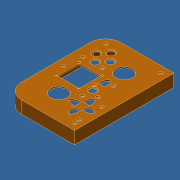
# Autodesk Inventor part: P1704_018_hautManette
Saved by Autodesk Inventor 2019 (Build 230136000, 136)
## iProperties
Created: 2019-05-28
Part Number: P1704_018_hautManette
Project: Nom Projet
Material: .
Description: Nom pièce
Document SubType Name: Modeling
Designer: Adel.KAHRIMANOVIC
Authority: brut Ø
Density: 0.001 g/cm^3
Appearance: Orange
Material number: ---
Author: Adel.KAHRIMANOVIC
Autodesk Inventor part; units mm, degrees
ref_plane "Plan YZ" through (0, 0, 0) normal (1, 0, 0) x (0, 1, 0)
ref_plane "Plan XZ" through (0, 0, 0) normal (0, 1, 0) x (-1, 0, 0)
ref_plane "Plan XY" through (0, 0, 0) normal (0, 0, 1) x (1, 0, 0)
sketch "Esquisse1" plane through (0, 0, 0) normal (0, 0, 1) x (1, 0, 0)
  line L0 (55, 80) -> (55, -80)
  line L1 (-55, -80) -> (-55, 80)
  line L2 (-55, 80) -> (55, -80) construction
  line L3 (55, 80) -> (-55, -80) construction
  line L4 (0, 0) -> (-55, 0) construction
  arc A0 (-55, -55) -> (-30, -80) centre (-30, -55) ccw
  line L5 (-30, -80) -> (55, -80)
  line L6 (-30, -80) -> (-30, -55) construction
  line L7 (55, 80) -> (-30, 80)
  arc A1 (-30, 80) -> (-55, 55) centre (-30, 55) ccw
  line L8 (-30, 55) -> (-30, 80) construction
  line L9 (-83.2132, 0) -> (78.0355, 0) projected
  line L10 (0, -119.2487) -> (0, 119.2487) projected
  dimension "d2" = 160
  dimension "d3" = 110
  dimension "d4" = 25
  dimension "d5" = 25
  constraints: 18 end point, 4 midpoint, 4 point on circle, 3 horizontal, 2 centre point, 2 parallel, 2 point on line, 2 tangent, 2 vertical, 1 collinear, 1 perpendicular
  measures "d2" distance of L0.start L0.end
  measures "d3" distance of L0.end L1.start
  measures "d4" distance of L5.start L6.end
  measures "d5" distance of L8.start L7.end
extrude "Extrusion1" add sketch "Esquisse1" along normal blind 22
sketch "Esquisse6" plane through (0, 0, 0) normal (0, 0, -1) x (-1, 0, 0)
  line L0 (-52.5, 77.5) -> (-52.5, -77.5)
  line L1 (-52.5, -77.5) -> (30, -77.5)
  line L2 (-52.5, 77.5) -> (30, 77.5)
  arc A0 (52.5, 55) -> (30, 77.5) centre (30, 55) ccw
  line L3 (52.5, 55) -> (52.5, -55)
  arc A1 (30, -77.5) -> (52.5, -55) centre (30, -55) ccw
  line L4 (-55, 80) -> (30, 80) projected
  line L5 (-55, -80) -> (-55, 80) projected
  line L6 (30, -80) -> (-55, -80) projected
  line L7 (55, 55) -> (55, -55) projected
  line L8 (30, -239.7653) -> (30, 84.7653) construction
  arc A2 (55, 55) -> (30, 80) centre (30, 55) ccw projected
  line L9 (-55, -80) -> (-55, 80) projected
  line L10 (30, -80) -> (-55, -80) projected
  arc A3 (30, -80) -> (55, -55) centre (30, -55) ccw projected
  line L11 (55, 55) -> (55, -55) projected
  arc A4 (55, 55) -> (30, 80) centre (30, 55) ccw projected
  line L12 (-55, 80) -> (30, 80) projected
  point P0 (0, 0)
  dimension "d8" = 2.5
  dimension "d9" = 2.5
  dimension "d10" = 2.5
  dimension "d11" = 2.5
  constraints: 10 end point, 4 point on circle, 4 tangent, 3 vertical, 2 centre point, 2 point on line, 1 horizontal, 1 midpoint, 1 perpendicular
  measures "d8" distance between parallel lines of L4 L2
  measures "d9" distance between parallel lines of L5 L0
  measures "d10" distance between parallel lines of L6 L1
  measures "d11" distance between parallel lines of L7 L3
extrude "Extrusion2" cut sketch "Esquisse6" against normal blind 2
sketch "Esquisse7" plane through (0, 0, 0) normal (0, 0, -1) x (-1, 0, 0)
  line L0 (-50, 75) -> (-50, -75)
  line L1 (-50, -75) -> (30, -75)
  line L2 (50, 55) -> (50, -55)
  line L3 (-50, 75) -> (30, 75)
  arc A0 (50, 55) -> (30, 75) centre (30, 55) ccw
  arc A1 (30, -75) -> (50, -55) centre (30, -55) ccw
  line L4 (30, 77.5) -> (-52.5, 77.5) projected
  line L5 (-52.5, 77.5) -> (-52.5, -77.5) projected
  line L6 (-52.5, -77.5) -> (30, -77.5) projected
  line L7 (52.5, -55) -> (52.5, 55) projected
  line L8 (30, 77.5) -> (30, 105.4816) construction
  point P0 (0, 0)
  dimension "d14" = 2.5
  dimension "d15" = 2.5
  dimension "d16" = 2.5
  dimension "d17" = 2.5
  constraints: 10 end point, 4 point on circle, 4 tangent, 3 vertical, 2 centre point, 2 point on line, 1 horizontal, 1 perpendicular
  measures "d14" distance between parallel lines of L3 L4
  measures "d15" distance between parallel lines of L5 L0
  measures "d16" distance between parallel lines of L6 L1
  measures "d17" distance between parallel lines of L7 L2
extrude "Extrusion3" cut sketch "Esquisse7" against normal blind 20
sketch "Esquisse8" plane through (0, 0, 22) normal (0, 0, 1) x (1, 0, 0)
  line L0 (-35, -17.5) -> (0, -17.5)
  line L1 (0, -17.5) -> (0, 17.5)
  line L2 (0, 17.5) -> (-35, 17.5)
  line L3 (-35, 17.5) -> (-35, -17.5)
  line L4 (-55, 55) -> (-55, -55) projected
  line L5 (-30, -80) -> (55, -80) projected
  line L6 (-13.2667, 17.5) -> (-13.2667, 80) construction
  line L7 (-17.5, -80) -> (-17.5, -17.5) construction
  line L8 (55, 80) -> (-30, 80) projected
  point P0 (0, 0)
  dimension "d20" = 35
  dimension "d21" = 35
  dimension "d24" = 20
  constraints: 12 end point, 3 parallel, 3 point on line, 2 vertical, 1 horizontal, 1 midpoint, 1 perpendicular
  measures "d20" distance of L2.end L0.start
  measures "d21" distance of L1.end L2.end
  measures "d24" distance between parallel lines of L4 L3
extrude "Extrusion4" cut sketch "Esquisse8" against normal through all
sketch "Esquisse9" plane through (0, 0, 22) normal (0, 0, 1) x (1, 0, 0)
  line L0 (-30, -75) -> (50, -75) projected
  line L1 (-50, 55) -> (-50, -55) projected
  point P0 (0, 0)
  point P1 (44.488, -68.904)
  dimension "d47" = 6.096
  dimension "d48" = 94.488
  measures "d47" distance from line of L0 point (44.488, -68.904)
  measures "d48" distance from line of L1 point (44.488, -68.904)
hole "Perçage1" at (44.488, -68.904, 22) direction (0, 0, -1) diameter 3.4 end through all countersink diameter 6.3 countersink angle 90
sketch "Esquisse10" plane through (0, 0, 22) normal (0, 0, 1) x (1, 0, 0)
  line L0 (-30, -75) -> (50, -75) projected
  line L1 (50, -75) -> (50, 75) projected
  line L2 (-50, 55) -> (-50, -55) projected
  point P0 (0, 0)
  point P1 (43.98, 69.78)
  dimension "d49" = 144.78
  dimension "d51" = 93.98
  measures "d49" distance from line of L0 point (43.98, 69.78)
  measures "d51" distance from line of point (43.98, 69.78) L2
hole "Perçage2" at (43.98, 69.78, 22) direction (0, 0, -1) diameter 3.4 end through all countersink diameter 6.3 countersink angle 90
sketch "Esquisse11" plane through (0, 0, 22) normal (0, 0, 1) x (1, 0, 0)
  line L0 (-30, -75) -> (50, -75) projected
  line L1 (-50, 55) -> (-50, -55) projected
  point P0 (0, 0)
  point P1 (-43.904, 1.2)
  dimension "d52" = 76.2
  dimension "d53" = 6.096
  measures "d52" distance from line of L0 point (-43.904, 1.2)
  measures "d53" distance from line of L1 point (-43.904, 1.2)
hole "Perçage3" at (-43.904, 1.2, 22) direction (0, 0, -1) diameter 3.4 end through all countersink diameter 6.3 countersink angle 90
sketch "Esquisse12" plane through (0, 0, 22) normal (0, 0, 1) x (1, 0, 0)
  circle A0 centre (-10, -40) radius 13.25
  line L0 (-30, -80) -> (55, -80) projected
  line L1 (-55, 55) -> (-55, -55) projected
  line L2 (-30, -75) -> (50, -75) projected
  line L3 (-50, 55) -> (-50, -55) projected
  circle A1 centre (15, 40) radius 13.25
  line L4 (50, -75) -> (50, 75) projected
  line L5 (50, 75) -> (-30, 75) projected
  point P0 (0, 0)
  dimension "d58" = 35
  dimension "d59" = 40
  dimension "d60" = 26.5
  dimension "d61" = 26.5
  dimension "d62" = 35
  dimension "d63" = 35
  constraints: 2 centre point
  measures "d58" distance from line of L2 A0.centre
  measures "d59" distance from line of A0.centre L3
  measures "d60" diameter of A0
  measures "d61" diameter of A1
  measures "d62" distance from line of L4 A1.centre
  measures "d63" distance from line of L5 A1.centre
extrude "Extrusion6" cut sketch "Esquisse12" against normal through all
sketch "Esquisse13" plane through (0, 0, 22) normal (0, 0, 1) x (1, 0, 0)
  line L0 (-30, -80) -> (55, -80) projected
  line L1 (-55, 55) -> (-55, -55) projected
  point P0 (0, 0)
  point P1 (-35.48, 45.24)
  dimension "d73" = 125.24
  dimension "d74" = 19.52
  measures "d73" distance from line of L0 point (-35.48, 45.24)
  measures "d74" distance from line of L1 point (-35.48, 45.24)
hole "Perçage4" at (-35.48, 45.24, 22) direction (0, 0, -1) diameter 11 end through all countersink diameter 13 countersink angle 90
sketch "Esquisse14" plane through (0, 0, 22) normal (0, 0, 1) x (1, 0, 0)
  line L0 (-30, -80) -> (55, -80) projected
  line L1 (-55, 55) -> (-55, -55) projected
  point P0 (0, 0)
  point P1 (-24.05, 32.535)
  dimension "d96" = 112.535
  dimension "d97" = 30.95
  measures "d96" distance from line of L0 point (-24.05, 32.535)
  measures "d97" distance from line of L1 point (-24.05, 32.535)
hole "Perçage5" at (-24.05, 32.535, 22) direction (0, 0, -1) diameter 11 end through all countersink diameter 13 countersink angle 90
sketch "Esquisse15" plane through (0, 0, 22) normal (0, 0, 1) x (1, 0, 0)
  line L0 (-30, -80) -> (55, -80) projected
  line L1 (-55, 55) -> (-55, -55) projected
  point P0 (0, 0)
  point P1 (-12.62, 45.24)
  dimension "d98" = 125.24
  dimension "d99" = 42.38
  measures "d98" distance from line of L0 point (-12.62, 45.24)
  measures "d99" distance from line of point (-12.62, 45.24) L1
hole "Perçage6" at (-12.62, 45.24, 22) direction (0, 0, -1) diameter 11 end through all countersink diameter 13 countersink angle 90
sketch "Esquisse16" plane through (0, 0, 22) normal (0, 0, 1) x (1, 0, 0)
  line L0 (-55, 55) -> (-55, -55) projected
  line L1 (-30, -80) -> (55, -80) projected
  point P0 (0, 0)
  point P1 (-24.05, 57.935)
  dimension "d100" = 30.95
  dimension "d101" = 137.935
  measures "d100" distance from line of L0 point (-24.05, 57.935)
  measures "d101" distance from line of L1 point (-24.05, 57.935)
hole "Perçage7" at (-24.05, 57.935, 22) direction (0, 0, -1) diameter 11 end through all countersink diameter 13 countersink angle 90
sketch "Esquisse17" plane through (0, 0, 22) normal (0, 0, 1) x (1, 0, 0)
  line L0 (-30, -80) -> (55, -80) projected
  line L1 (55, -80) -> (55, 80) projected
  point P0 (0, 0)
  point P1 (13.128, -8.826)
  dimension "d109" = 71.174
  dimension "d110" = 41.872
  measures "d109" distance from line of L0 point (13.128, -8.826)
  measures "d110" distance from line of L1 point (13.128, -8.826)
hole "Perçage8" at (13.128, -8.826, 22) direction (0, 0, -1) diameter 11 end through all countersink diameter 13 countersink angle 90
sketch "Esquisse18" plane through (0, 0, 22) normal (0, 0, 1) x (1, 0, 0)
  line L0 (-30, -80) -> (55, -80) projected
  line L1 (55, -80) -> (55, 80) projected
  ellipse E0 centre (21.12, -40.235) end of major axis (34.77, -40.235) minor radius 5.5
  line L2 (21.12, -34.735) -> (21.12, -45.735)
  line L3 (7.47, -35.359) -> (7.47, -41.6011) construction
  line L4 (15.3478, -40.235) -> (31.1531, -40.235) construction
  point P0 (0, 0)
  point P1 (33.374, -40.235)
  point P2 (15.62, -40.235)
  dimension "d135" = 13.65
  dimension "d133" = 11
  dimension "d136" = 13.65
  dimension "d142" = 5.5
  dimension "d143" = 39.765
  dimension "d144" = 39.38
  constraints: 6 end point, 3 vertical, 2 midpoint, 2 point on line, 1 horizontal, 4 other
  measures "d133" distance of L2.start L2.end
  measures "d136" distance between parallel lines of L3 L2
  measures "d142" distance from line of point (15.62, -40.235) L2
  measures "d143" distance from line of L0 point (15.62, -40.235)
  measures "d144" distance from line of L1 point (15.62, -40.235)
extrude "Extrusion7" cut sketch "Esquisse18" against normal blind 10 contours L2 E0 picked at (17.5726, -38.6005)
sketch "Esquisse19" plane through (0, 0, 22) normal (0, 0, 1) x (1, 0, 0)
  line L0 (32.98, -34.735) -> (32.98, -45.735)
  ellipse E0 centre (32.98, -40.235) end of major axis (32.98, -34.735) minor radius 13.65
  line L1 (35.2239, -40.235) -> (43.4479, -40.235) construction
  line L2 (55, -80) -> (55, 80) projected
  line L3 (-30, -80) -> (55, -80) projected
  point P0 (0, 0)
  point P1 (38.48, -40.235)
  dimension "d148" = 13.65
  dimension "d147" = 11
  dimension "d150" = 5.5
  dimension "d151" = 16.52
  dimension "d152" = 39.765
  constraints: 4 end point, 2 midpoint, 2 point on line, 1 horizontal, 1 vertical, 4 other
  measures "d147" distance of L0.start L0.end
  measures "d150" distance from line of point (38.48, -40.235) L0
  measures "d151" distance from line of L2 point (38.48, -40.235)
  measures "d152" distance from line of L3 point (38.48, -40.235)
extrude "Extrusion8" cut sketch "Esquisse19" against normal blind 10 contours E0 L0 picked at (36.5274, -41.8695)
sketch "Esquisse20" plane through (0, 0, 22) normal (0, 0, 1) x (1, 0, 0)
  ellipse E0 centre (27.05, -33.035) end of major axis (32.55, -33.035) minor radius 13.65
  line L0 (32.55, -33.035) -> (21.55, -33.035)
  line L1 (27.05, -22.7093) -> (27.05, -43.3607) construction
  line L2 (55, -80) -> (55, 80) projected
  line L3 (-30, -80) -> (55, -80) projected
  point P0 (0, 0)
  point P1 (27.05, -27.535)
  dimension "d156" = 13.65
  dimension "d155" = 11
  dimension "d157" = 5.5
  dimension "d158" = 27.95
  dimension "d159" = 52.465
  constraints: 4 end point, 3 midpoint, 1 horizontal, 1 point on line, 1 vertical, 4 other
  measures "d155" distance of L0.start L0.end
  measures "d157" distance from line of point (27.05, -27.535) L0
  measures "d158" distance from line of L2 point (27.05, -27.535)
  measures "d159" distance from line of L3 point (27.05, -27.535)
extrude "Extrusion9" cut sketch "Esquisse20" against normal blind 10 contours E0 L0 picked at (28.6816, -29.7706)
sketch "Esquisse21" plane through (0, 0, 22) normal (0, 0, 1) x (1, 0, 0)
  ellipse E0 centre (27.05, -47.435) end of major axis (21.55, -47.435) minor radius 13.65
  line L0 (21.55, -47.435) -> (32.55, -47.435)
  line L1 (27.05, -58.4489) -> (27.05, -51.8094) construction
  line L2 (-30, -80) -> (55, -80) projected
  line L3 (55, -80) -> (55, 80) projected
  point P0 (0, 0)
  point P1 (27.05, -52.935)
  dimension "d163" = 13.65
  dimension "d162" = 11
  dimension "d164" = 5.5
  dimension "d165" = 27.065
  dimension "d166" = 27.95
  constraints: 4 end point, 2 midpoint, 2 point on line, 1 horizontal, 1 vertical, 4 other
  measures "d162" distance of L0.start L0.end
  measures "d164" distance from line of point (27.05, -52.935) L0
  measures "d165" distance from line of L2 point (27.05, -52.935)
  measures "d166" distance from line of L3 point (27.05, -52.935)
extrude "Extrusion10" cut sketch "Esquisse21" against normal blind 10 contours E0 L0 picked at (25.4184, -50.6994)
sketch "Esquisse22" plane through (0, 0, 22) normal (0, 0, 1) x (1, 0, 0)
  ellipse E0 centre (13.158, 5.358) end of major axis (18.658, 5.358) minor radius 13.65
  line L0 (7.658, 5.358) -> (18.658, 5.358)
  line L1 (13.158, 8.3674) -> (13.158, 2.3486) construction
  line L2 (55, -80) -> (55, 80) projected
  line L3 (55, 80) -> (-30, 80) projected
  point P0 (0, 0)
  point P1 (13.158, 10.858)
  dimension "d174" = 13.65
  dimension "d173" = 11
  dimension "d175" = 5.5
  dimension "d176" = 41.842
  dimension "d177" = 69.142
  constraints: 4 end point, 3 midpoint, 1 horizontal, 1 point on line, 1 vertical, 4 other
  measures "d173" distance of L0.start L0.end
  measures "d175" distance from line of L0 point (13.158, 10.858)
  measures "d176" distance from line of L2 point (13.158, 10.858)
  measures "d177" distance from line of L3 point (13.158, 10.858)
extrude "Extrusion11" cut sketch "Esquisse22" against normal blind 10 contours E0 L0 picked at (14.7896, 8.6224)
sketch "Esquisse23" plane through (0, 0, 22) normal (0, 0, 1) x (1, 0, 0)
  line L0 (-30, -80) -> (55, -80) projected
  line L1 (55, -80) -> (55, 80) projected
  point P0 (0, 0)
  point P1 (43.56, -24.995)
  dimension "d187" = 55.005
  dimension "d188" = 11.44
  measures "d187" distance from line of L0 point (43.56, -24.995)
  measures "d188" distance from line of L1 point (43.56, -24.995)
hole "Perçage9" at (43.56, -24.995, 22) direction (0, 0, -1) diameter 3.4 end through all countersink diameter 6.3 countersink angle 90
pattern_linear "Réseau rectangulaire1" count 2 spacing 35.56 along (0, -1, 0) of "Perçage9"
pattern_linear "Réseau rectangulaire2" count 2 spacing 30.48 along (-1, 0, 0) of "Perçage9"
sketch "Esquisse24" plane through (0, 0, 22) normal (0, 0, 1) x (1, 0, 0)
  line L0 (-55, 55) -> (-55, -55) projected
  line L1 (55, 80) -> (-30, 80) projected
  point P0 (0, 0)
  point P1 (-40.56, 29.995)
  dimension "d205" = 14.44
  dimension "d206" = 50.005
  measures "d205" distance from line of L0 point (-40.56, 29.995)
  measures "d206" distance from line of L1 point (-40.56, 29.995)
hole "Perçage10" at (-40.56, 29.995, 22) direction (0, 0, -1) diameter 3.4 end through all countersink diameter 6.3 countersink angle 90
pattern_linear "Réseau rectangulaire3" count 2 spacing 30.48 along (1, 0, 0) of "Perçage10"
pattern_linear "Réseau rectangulaire4" count 2 spacing 35.56 along (0, 1, 0) of "Perçage10"
sketch "Esquisse25" plane through (0, 0, 22) normal (0, 0, 1) x (1, 0, 0)
  line L0 (55, -80) -> (55, 80) projected
  line L1 (-30, -80) -> (55, -80) projected
  point P0 (0, 0)
  point P1 (27.352, -14.033)
  dimension "d220" = 27.648
  dimension "d221" = 65.967
  measures "d220" distance from line of L0 point (27.352, -14.033)
  measures "d221" distance from line of L1 point (27.352, -14.033)
hole "Perçage11" at (27.352, -14.033, 22) direction (0, 0, -1) diameter 3.4 end through all countersink diameter 6.3 countersink angle 90
sketch "Esquisse26" plane through (0, 0, 22) normal (0, 0, 1) x (1, 0, 0)
  line L0 (55, -80) -> (55, 80) projected
  line L1 (-30, -80) -> (55, -80) projected
  point P0 (0, 0)
  point P1 (23.923, 14.034)
  dimension "d229" = 31.077
  dimension "d230" = 94.034
  measures "d229" distance from line of L0 point (23.923, 14.034)
  measures "d230" distance from line of L1 point (23.923, 14.034)
hole "Perçage12" at (23.923, 14.034, 22) direction (0, 0, -1) diameter 3.4 end through all countersink diameter 6.3 countersink angle 90
sketch "Esquisse27" plane through (0, 0, 22) normal (0, 0, 1) x (1, 0, 0)
  line L0 (55, -80) -> (55, 80) projected
  line L1 (-30, -80) -> (55, -80) projected
  point P0 (0, 0)
  point P1 (7.794, -0.19)
  dimension "d238" = 47.206
  dimension "d239" = 79.81
  measures "d238" distance from line of L0 point (7.794, -0.19)
  measures "d239" distance from line of L1 point (7.794, -0.19)
hole "Perçage13" at (7.794, -0.19, 22) direction (0, 0, -1) diameter 3.4 end through all countersink diameter 6.3 countersink angle 90
sketch "Esquisse28" plane through (0, 0, 22) normal (0, 0, 1) x (1, 0, 0)
  line L0 (55, -80) -> (55, 80) projected
  line L1 (-30, -80) -> (55, -80) projected
  point P0 (0, 0)
  point P1 (0.94, -19.015)
  dimension "d247" = 54.06
  dimension "d248" = 60.985
  measures "d247" distance from line of L0 point (0.94, -19.015)
  measures "d248" distance from line of L1 point (0.94, -19.015)
hole "Perçage14" at (0.94, -19.015, 22) direction (0, 0, -1) diameter 2.9 end through all countersink diameter 3.5 countersink angle 90
pattern_linear "Réseau rectangulaire5" count 2 spacing 38.1 along (0, 1, 0) count 2 spacing 36.9 along (-1, 0, 0) of "Perçage14"
